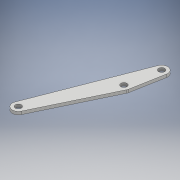
# Autodesk Inventor part: 三角塊3
Saved by Autodesk Inventor 2017 (Build 210142000, 142)
## iProperties
Part Number: 三角塊3
Material: 一般
Document SubType Name: Modeling
Designer: user
Density: 1 g/cm^3
Appearance: 預設
Author: user
Autodesk Inventor part; units mm, degrees
ref_plane "YZ Plane" through (0, 0, 0) normal (1, 0, 0) x (0, 1, 0)
ref_plane "XZ Plane" through (0, 0, 0) normal (0, 1, 0) x (-1, 0, 0)
ref_plane "XY Plane" through (0, 0, 0) normal (0, 0, 1) x (1, 0, 0)
sketch "草圖1" plane through (0, 0, 0) normal (0, 0, 1) x (1, 0, 0)
  line L0 (0, 0) -> (13.2614, 34.1988)
  line L1 (11.3356, 23.643) -> (10.4709, 21.8396)
  line L2 (11.3967, 34.9219) -> (-1.8647, 0.7231)
  line L3 (13.255, 23.0202) -> (1.8034, -0.8647)
  line L4 (13.2272, 22.8679) -> (15.2289, 33.8398)
  arc A0 (13.139, 22.7784) -> (13.3031, 23.2841) centre (11.3356, 23.643) ccw
  arc A1 (15.2289, 33.8398) -> (11.3967, 34.9219) centre (13.2614, 34.1988) ccw
  arc A2 (12.5383, 32.3341) -> (12.9025, 32.2313) centre (13.2614, 34.1988) ccw
  arc A3 (0.8647, 1.8034) -> (0.7231, 1.8647) centre (0, 0) ccw
  arc A4 (-1.8647, 0.7231) -> (1.8034, -0.8647) centre (0, 0) ccw
  dimension "d0" = 10.73
  dimension "d1" = 26.22
  dimension "d2" = 36.68
  constraints: 10 end point, 10 point on circle, 6 tangent, 5 centre point, 5 point on line, 3 coincident
  measures "d0" distance of L0.end L1.start
  measures "d1" distance of L1.start L0.start
  measures "d2" distance of L0.start L0.end
extrude "擠出1" add sketch "草圖1" along normal blind 1 contours A1 L4 A0 L3 A4 L2
sketch "草圖2" plane through (0, 0, 1) normal (0, 0, 1) x (1, 0, 0)
  arc A0 (13.139, 22.7784) -> (13.3031, 23.2841) centre (11.3356, 23.643) ccw projected
  circle A1 centre (11.3356, 23.643) radius 1
  arc A2 (15.2289, 33.8398) -> (11.3967, 34.9219) centre (13.2614, 34.1988) ccw projected
  circle A3 centre (13.2614, 34.1988) radius 1
  arc A4 (-1.8647, 0.7231) -> (1.8034, -0.8647) centre (0, 0) ccw projected
  circle A5 centre (0, 0) radius 1
  dimension "d8" = 2
  dimension "d9" = 2
  dimension "d10" = 2
  constraints: 3 centre point, 3 coincident
  measures "d8" diameter of A1
  measures "d9" diameter of A5
  measures "d10" diameter of A3
extrude "擠出2" cut sketch "草圖2" against normal blind 10
